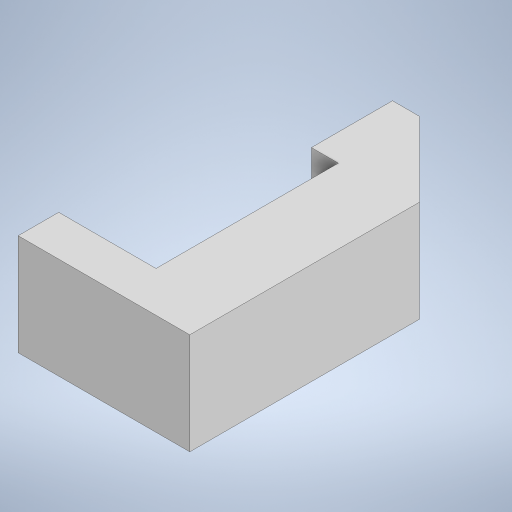
# Autodesk Inventor part: focus mount
Saved by Autodesk Inventor 2024 (Build 280153000, 153)
## iProperties
Created: 2025-05-22
Part Number: focus mount
Material: Generic
Document SubType Name: Modeling
Designer: Williamow
Density: 1 g/cm^3
Appearance: Default
Author: Williamow
Autodesk Inventor part; units mm, degrees
ref_plane "YZ Plane" through (0, 0, 0) normal (1, 0, 0) x (0, 1, 0)
ref_plane "XZ Plane" through (0, 0, 0) normal (0, 1, 0) x (-1, 0, 0)
ref_plane "XY Plane" through (0, 0, 0) normal (0, 0, 1) x (1, 0, 0)
sketch "Sketch1" plane through (0, 0, 0) normal (0, 1, 0) x (-1, 0, 0)
  line L0 (0, 0) -> (0, -34)
  line L1 (0, -34) -> (11, -45)
  line L2 (11, -45) -> (15, -45)
  line L3 (15, -45) -> (15, -33)
  line L4 (6.7118, 0) -> (0, 0)
  line L5 (15, -33) -> (11, -33)
  line L6 (11, -33) -> (11, -6)
  line L7 (11, -6) -> (25.4, -6)
  line L8 (25.4, -6) -> (25.4, 0)
  line L9 (25.4, 0) -> (6.7118, 0)
  dimension "d0" = 135
  dimension "d1" = 15
  dimension "d2" = 4
  dimension "d13" = 4
  dimension "d14" = 25.4
  dimension "d15" = 6
  dimension "d16" = 12
  dimension "d17" = 45
  constraints: 20 end point, 7 perpendicular, 1 horizontal, 1 vertical
  measures "d0" angle of L0 L1
  measures "d1" horizontal distance of L0.end L2.end
  measures "d2" distance of L1.end L2.end
  measures "d13" distance of L3.end L5.end
  measures "d14" distance of L0.start L8.end
  measures "d15" distance of L7.end L8.end
  measures "d16" distance of L2.end L3.end
  measures "d17" vertical distance of L8.end L2.end
extrude "Extrusion1" add sketch "Sketch1" along normal mid plane 15
sketch "Sketch2" plane through (-15, -7.5, 0) normal (-1, 0, 0) x (0, 0, 1)
  line L0 (-45, 0) -> (-45, 15) projected
  circle A0 centre (-39, 7.5) radius 4.0005
  point P0 (0, 7.5)
  point P1 (-45, 7.5)
  dimension "d6" = 6
  dimension "d7" = 8.001
  constraints: 1 centre point, 1 horizontal alignment, 1 midpoint
  measures "d6" distance from line of L0 A0.centre
  measures "d7" diameter of A0
extrude "Extrusion2" cut sketch "Sketch2" against normal through all
sketch "Sketch3" plane through (-11, 7.5, -45) normal (0, 0, -1) x (-1, 0, 0)
  line L0 (4, -15) -> (4, 0) projected
  line L1 (4, -15) -> (0, -15) projected
  circle A0 centre (2, -7.5) radius 0.6
  point P0 (-11, -7.5)
  point P1 (2, -15)
  point P2 (4, -7.5)
  dimension "d10" = 1.2
  constraints: 2 midpoint, 1 centre point, 1 horizontal alignment, 1 vertical alignment
  measures "d10" diameter of A0
extrude "Extrusion3" cut sketch "Sketch3" against normal up to next
body "Solid1"
